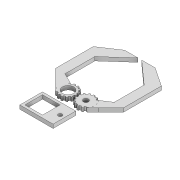
# Autodesk Inventor part: Gripper_dentado
Saved by Autodesk Inventor 2021 (Build 250183000, 183)
## iProperties
Created: 2022-06-07
Part Number: Gripper_dentado
Material: Genérico
Document SubType Name: Modeling
Designer: orgyn
Density: 1 g/cm^3
Appearance: Valor por defecto
Author: orgyn
Autodesk Inventor part; units mm, degrees
ref_plane "YZ Plane" through (0, 0, 0) normal (1, 0, 0) x (0, 1, 0)
ref_plane "XZ Plane" through (0, 0, 0) normal (0, 1, 0) x (-1, 0, 0)
ref_plane "XY Plane" through (0, 0, 0) normal (0, 0, 1) x (1, 0, 0)
sketch "Boceto1" plane through (0, 0, 0) normal (0, 1, 0) x (-1, 0, 0)
  line L0 (6.9821, 0.4997) -> (6.9821, -0.4997)
  line L1 (5.9531, 0.7485) -> (6.9821, 0.4997)
  line L2 (5.9531, -0.7485) -> (6.9821, -0.4997)
  line L3 (5.0388, 3.2574) -> (6.0739, 3.4796)
  line L4 (5.6884, 1.9086) -> (6.5075, 2.5792)
  line L5 (6.0739, 3.4796) -> (6.5075, 2.5792)
  line L6 (3.1265, 5.121) -> (3.9626, 5.7704)
  line L7 (4.2969, 4.1876) -> (4.744, 5.1473)
  line L8 (3.9626, 5.7704) -> (4.744, 5.1473)
  line L9 (0.5949, 5.9704) -> (1.0665, 6.9183)
  line L10 (2.0545, 5.6373) -> (2.0408, 6.6959)
  line L11 (1.0665, 6.9183) -> (2.0408, 6.6959)
  line L12 (-2.0545, 5.6373) -> (-2.0408, 6.6959)
  line L13 (-0.5949, 5.9704) -> (-1.0665, 6.9183)
  line L14 (-2.0408, 6.6959) -> (-1.0665, 6.9183)
  line L15 (-4.2969, 4.1876) -> (-4.744, 5.1473)
  line L16 (-3.1265, 5.121) -> (-3.9626, 5.7704)
  line L17 (-4.744, 5.1473) -> (-3.9626, 5.7704)
  line L18 (-5.6884, 1.9086) -> (-6.5075, 2.5792)
  line L19 (-5.0388, 3.2574) -> (-6.0739, 3.4796)
  line L20 (-6.5075, 2.5792) -> (-6.0739, 3.4796)
  line L21 (-5.9531, -0.7485) -> (-6.9821, -0.4997)
  line L22 (-5.9531, 0.7485) -> (-6.9821, 0.4997)
  line L23 (-6.9821, -0.4997) -> (-6.9821, 0.4997)
  line L24 (-5.0388, -3.2574) -> (-6.0739, -3.4796)
  line L25 (-5.6884, -1.9086) -> (-6.5075, -2.5792)
  line L26 (-6.0739, -3.4796) -> (-6.5075, -2.5792)
  line L27 (-3.1265, -5.121) -> (-3.9626, -5.7704)
  line L28 (-4.2969, -4.1876) -> (-4.744, -5.1473)
  line L29 (-3.9626, -5.7704) -> (-4.744, -5.1473)
  line L30 (-0.5949, -5.9704) -> (-1.0665, -6.9183)
  line L31 (-2.0545, -5.6373) -> (-2.0408, -6.6959)
  line L32 (-1.0665, -6.9183) -> (-2.0408, -6.6959)
  line L33 (2.0545, -5.6373) -> (2.0408, -6.6959)
  line L34 (0.5949, -5.9704) -> (1.0665, -6.9183)
  line L35 (2.0408, -6.6959) -> (1.0665, -6.9183)
  line L36 (4.2969, -4.1876) -> (4.744, -5.1473)
  line L37 (3.1265, -5.121) -> (3.9626, -5.7704)
  line L38 (4.744, -5.1473) -> (3.9626, -5.7704)
  line L39 (5.6884, -1.9086) -> (6.5075, -2.5792)
  line L40 (5.0388, -3.2574) -> (6.0739, -3.4796)
  line L41 (6.5075, -2.5792) -> (6.0739, -3.4796)
  arc A0 (6.5075, 2.5792) -> (6.0739, 3.4796) centre (0, 0) ccw
  arc A1 (4.744, 5.1473) -> (3.9626, 5.7704) centre (0, 0) ccw
  arc A2 (5.9531, 0.7485) -> (5.6884, 1.9086) centre (0, 0) ccw
  arc A3 (5.6884, -1.9086) -> (5.9531, -0.7485) centre (0, 0) ccw
  arc A4 (4.2969, -4.1876) -> (5.0388, -3.2574) centre (0, 0) ccw
  arc A5 (3.9626, -5.7704) -> (4.744, -5.1473) centre (0, 0) ccw
  arc A6 (2.0545, -5.6373) -> (3.1265, -5.121) centre (0, 0) ccw
  arc A7 (1.0665, -6.9183) -> (2.0408, -6.6959) centre (0, 0) ccw
  arc A8 (-0.5949, -5.9704) -> (0.5949, -5.9704) centre (0, 0) ccw
  arc A9 (-2.0408, -6.6959) -> (-1.0665, -6.9183) centre (0, 0) ccw
  arc A10 (-3.1265, -5.121) -> (-2.0545, -5.6373) centre (0, 0) ccw
  arc A11 (-4.744, -5.1473) -> (-3.9626, -5.7704) centre (0, 0) ccw
  arc A12 (-5.0388, -3.2574) -> (-4.2969, -4.1876) centre (0, 0) ccw
  arc A13 (-6.5075, -2.5792) -> (-6.0739, -3.4796) centre (0, 0) ccw
  arc A14 (-5.9531, -0.7485) -> (-5.6884, -1.9086) centre (0, 0) ccw
  arc A15 (-6.9821, 0.4997) -> (-6.9821, -0.4997) centre (0, 0) ccw
  arc A16 (-5.6884, 1.9086) -> (-5.9531, 0.7485) centre (0, 0) ccw
  arc A17 (-6.0739, 3.4796) -> (-6.5075, 2.5792) centre (0, 0) ccw
  arc A18 (-4.2969, 4.1876) -> (-5.0388, 3.2574) centre (0, 0) ccw
  arc A19 (-3.9626, 5.7704) -> (-4.744, 5.1473) centre (0, 0) ccw
  arc A20 (-2.0545, 5.6373) -> (-3.1265, 5.121) centre (0, 0) ccw
  arc A21 (2.0408, 6.6959) -> (1.0665, 6.9183) centre (0, 0) ccw
  arc A22 (-1.0665, 6.9183) -> (-2.0408, 6.6959) centre (0, 0) ccw
  arc A23 (0.5949, 5.9704) -> (-0.5949, 5.9704) centre (0, 0) ccw
  arc A24 (5.0388, 3.2574) -> (4.2969, 4.1876) centre (0, 0) ccw
  arc A25 (3.1265, 5.121) -> (2.0545, 5.6373) centre (0, 0) ccw
  circle A26 centre (0, 0) radius 4.5
  line L42 (-7, 0) -> (-7.2, 0)
  line L43 (-7.2, 0) -> (-21.2, 0)
  line L44 (-7.5804, 2.2898) -> (-7.3217, 1.3245)
  line L45 (-8.6387, 2.2638) -> (-7.5804, 2.2898)
  line L46 (-8.2513, 0.8178) -> (-7.3217, 1.3245)
  line L47 (-10.1712, 4.4505) -> (-9.229, 4.9331)
  line L48 (-9.1947, 3.3158) -> (-8.5771, 4.1756)
  line L49 (-9.229, 4.9331) -> (-8.5771, 4.1756)
  line L50 (-12.5008, 5.7557) -> (-11.8612, 6.5994)
  line L51 (-11.1286, 5.1571) -> (-10.9452, 6.1998)
  line L52 (-11.8612, 6.5994) -> (-10.9452, 6.1998)
  line L53 (-15.1659, 5.921) -> (-14.9557, 6.9586)
  line L54 (-13.6699, 5.977) -> (-13.957, 6.9959)
  line L55 (-17.6388, 4.9135) -> (-17.8996, 5.9395)
  line L56 (-16.3152, 5.613) -> (-17.016, 6.4065)
  line L57 (-19.4297, 2.9328) -> (-20.1098, 3.7441)
  line L58 (-18.5407, 4.1374) -> (-19.5164, 4.5482)
  line L59 (-20.1098, 3.7441) -> (-19.5164, 4.5482)
  line L60 (-20.1838, 0.3713) -> (-21.1486, 0.8071)
  line L61 (-19.9055, 1.8422) -> (-20.9628, 1.789)
  line L62 (-21.1486, 0.8071) -> (-20.9628, 1.789)
  line L63 (-19.7518, -2.2638) -> (-20.8102, -2.2898)
  line L64 (-20.1393, -0.8178) -> (-21.0688, -1.3245)
  line L65 (-20.8102, -2.2898) -> (-21.0688, -1.3245)
  line L66 (-18.2193, -4.4505) -> (-19.1616, -4.9331)
  line L67 (-19.1958, -3.3158) -> (-19.8135, -4.1756)
  line L68 (-19.1616, -4.9331) -> (-19.8135, -4.1756)
  line L69 (-15.8898, -5.7557) -> (-16.5294, -6.5994)
  line L70 (-17.262, -5.1571) -> (-17.4454, -6.1998)
  line L71 (-16.5294, -6.5994) -> (-17.4454, -6.1998)
  line L72 (-13.2247, -5.921) -> (-13.4349, -6.9586)
  line L73 (-14.7207, -5.977) -> (-14.4336, -6.9959)
  line L74 (-13.4349, -6.9586) -> (-14.4336, -6.9959)
  line L75 (-10.7518, -4.9135) -> (-10.491, -5.9395)
  line L76 (-12.0754, -5.613) -> (-11.3745, -6.4065)
  line L77 (-10.491, -5.9395) -> (-11.3745, -6.4065)
  line L78 (-8.9609, -2.9328) -> (-8.2808, -3.7441)
  line L79 (-9.8499, -4.1374) -> (-8.8742, -4.5482)
  line L80 (-8.2808, -3.7441) -> (-8.8742, -4.5482)
  line L81 (-8.2068, -0.3713) -> (-7.242, -0.8071)
  line L82 (-8.4851, -1.8422) -> (-7.4278, -1.789)
  line L83 (-7.242, -0.8071) -> (-7.4278, -1.789)
  arc A27 (-8.5771, 4.1756) -> (-9.229, 4.9331) centre (-14.1953, 0) ccw
  arc A28 (-10.9452, 6.1998) -> (-11.8612, 6.5994) centre (-14.1953, 0) ccw
  arc A29 (-8.6387, 2.2638) -> (-9.1947, 3.3158) centre (-14.1953, 0) ccw
  arc A30 (-8.2068, -0.3713) -> (-8.2513, 0.8178) centre (-14.1953, 0) ccw
  arc A31 (-7.4278, -1.789) -> (-7.242, -0.8071) centre (-14.1953, 0) ccw
  arc A32 (-8.9609, -2.9328) -> (-8.4851, -1.8422) centre (-14.1953, 0) ccw
  arc A33 (-8.8742, -4.5482) -> (-8.2808, -3.7441) centre (-14.1953, 0) ccw
  arc A34 (-10.7518, -4.9135) -> (-9.8499, -4.1374) centre (-14.1953, 0) ccw
  arc A35 (-11.3745, -6.4065) -> (-10.491, -5.9395) centre (-14.1953, 0) ccw
  arc A36 (-13.2247, -5.921) -> (-12.0754, -5.613) centre (-14.1953, 0) ccw
  arc A37 (-14.4336, -6.9959) -> (-13.4349, -6.9586) centre (-14.1953, 0) ccw
  arc A38 (-15.8898, -5.7557) -> (-14.7207, -5.977) centre (-14.1953, 0) ccw
  arc A39 (-17.4454, -6.1998) -> (-16.5294, -6.5994) centre (-14.1953, 0) ccw
  arc A40 (-18.2193, -4.4505) -> (-17.262, -5.1571) centre (-14.1953, 0) ccw
  arc A41 (-19.8135, -4.1756) -> (-19.1616, -4.9331) centre (-14.1953, 0) ccw
  arc A42 (-19.7518, -2.2638) -> (-19.1958, -3.3158) centre (-14.1953, 0) ccw
  arc A43 (-21.0688, -1.3245) -> (-20.8102, -2.2898) centre (-14.1953, 0) ccw
  arc A44 (-20.1838, 0.3713) -> (-20.1393, -0.8178) centre (-14.1953, 0) ccw
  arc A45 (-20.9628, 1.789) -> (-21.1486, 0.8071) centre (-14.1953, 0) ccw
  arc A46 (-19.4297, 2.9328) -> (-19.9055, 1.8422) centre (-14.1953, 0) ccw
  arc A47 (-19.5164, 4.5482) -> (-20.1098, 3.7441) centre (-14.1953, 0) ccw
  arc A48 (-17.6388, 4.9135) -> (-18.5407, 4.1374) centre (-14.1953, 0) ccw
  arc A49 (-13.957, 6.9959) -> (-14.9557, 6.9586) centre (-14.1953, 0) ccw
  arc A50 (-17.016, 6.4065) -> (-17.8996, 5.9395) centre (-14.1953, 0) ccw
  arc A51 (-15.1659, 5.921) -> (-16.3152, 5.613) centre (-14.1953, 0) ccw
  arc A52 (-10.1712, 4.4505) -> (-11.1286, 5.1571) centre (-14.1953, 0) ccw
  arc A53 (-12.5008, 5.7557) -> (-13.6699, 5.977) centre (-14.1953, 0) ccw
  circle A54 centre (-14.1953, 0) radius 2
  line L84 (0, 0) -> (-2, 0)
  line L85 (-2, 0) -> (2, 0)
  line L86 (-14.1953, 0) -> (-16.1953, 0)
  line L87 (0, 0) -> (20, 0)
  line L88 (0, 0) -> (10, 0)
  line L89 (20, -10) -> (10, 0)
  line L90 (20, -40) -> (5, -50)
  line L91 (12.5, -33.8004) -> (12.5, -10)
  line L92 (12.5, -10) -> (4.0311, -2)
  line L93 (10, 0) -> (4.744, 5.1473)
  line L94 (20, -39.7931) -> (20, -10)
  line L95 (12.5, -33.8004) -> (-5.5976, -50)
  line L96 (-34.1953, -10) -> (-24.1953, 0)
  line L97 (-34.1953, -40) -> (-19.1953, -50)
  line L98 (-26.6953, -33.8004) -> (-26.6953, -10)
  line L99 (-24.1953, 0) -> (-19.2423, 4.8505)
  line L100 (-34.1953, -39.7931) -> (-34.1953, -10)
  line L101 (-26.6953, -33.8004) -> (-8.5976, -50)
  line L102 (-26.6953, -10) -> (-18.2193, -4.4505)
  line L103 (-19.3535, -3.0647) -> (-19.0804, -2.8067)
  line L104 (-18.5981, -2.3512) -> (-18.4725, -2.2324)
  line L105 (-18.3019, -2.0713) -> (-18.2264, -2)
  line L106 (5, -50) -> (-5.5976, -50)
  line L107 (-8.5976, -50) -> (-19.1953, -50)
  circle A55 centre (0, 0) radius 4.5
  line L108 (10, 0) -> (4.5, 0)
  line L109 (5.9249, -3.789) -> (8.4708, 1.4976)
  line L110 (5.9249, -3.789) -> (12.5, -10)
  line L111 (12.5, -10) -> (12.5, -33.8004)
  line L112 (12.5, -33.8004) -> (-5.5976, -50)
  line L113 (-5.5976, -50) -> (5, -50)
  line L114 (20, -39.7931) -> (20, -40)
  line L115 (-34.1953, -40) -> (-34.1953, -39.7931)
  line L116 (-19.5164, 4.5482) -> (-19.5334, 4.5655)
  line L117 (12.5, -10) -> (3.9626, -5.7704)
  point P0 (-20.9568, -1.8117)
  point P1 (-18.9393, 5.1473)
  point P2 (5.4573, -3.3472)
  dimension "d14" = 4
  dimension "d6" = 360
  dimension "d9" = 0.2
  dimension "d15" = 2
  dimension "d16" = 4
  constraints: 236 end point, 110 point on circle, 53 centre point, 13 point on line, 5 coincident, 5 horizontal, 3 equal length, 2 horizontal alignment, 2 perpendicular, 2 vertical, 1 midpoint, 106 other
  measures "d9" distance of L42.start L42.end
  measures "d15" distance of L84.start L84.end
  measures "d16" distance of L84.end L85.end
extrude "Extrusión1" add sketch "Boceto1" along normal blind 3 contours L1 A2 L4 A0 L3 A24 L7 L93 L109 L87 L0 | L0 L87 A26 L92 L40 A4 L36 L38 L37 A6 L33 L35 L34 A8 L30 L32 L31 A10 L27 L29 L28 A12 L24 L26 L25 A14 L21 L23 L22 A16 L18 L20 L19 A18 L15 L17 L16 A20 L12 L14 L13 A23 L9 L11 L10 A25 L6 L8 L7 A24 L3 L5 L4 A2 L1 | L87 L109 L39 A3 L2 L0 | L0 L2 A3 L39 L41 L40 L92 A26 L87 | L109 L93 L87 | L87 L89 L94 L114 L90 L106 L95 L91 L92 L109 L41 | A30 L81 L83 L82 A32 L78 L80 L79 A34 L75 L77 L76 A36 L72 L74 L73 A38 L69 L71 L70 A40 L66 L68 L67 A42 L63 L65 L64 A44 L43 A54 | L43 A54 A44 L60 L62 L61 A46 L57 L59 L58 A48 L55 A50 L56 A51 L53 A49 L54 A53 L50 L52 L51 A52 L47 L49 L48 A29 L45 L44 L46 A30 | L92 L117 A5 L36 A4 L40 | L40 L109 L92 | A44 L64 A43 L63 A42 L67 A41 L66 L102 L98 L101 L107 L97 L115 L100 L96 L99 L116 A47 L57 A46 L61 A45 L60
sketch "Boceto2" plane through (0, 0, 0) normal (0, -1, 0) x (1, 0, 0)
  line L0 (0, 0) -> (0, 20.3173)
  line L1 (0, 20.3173) -> (14, 20.3173)
  line L2 (0, 20.3173) -> (0, 13.3173)
  line L3 (0, 13.3173) -> (-7, 13.3173)
  line L4 (-7, 13.3173) -> (-7, 27.3173)
  line L5 (-7, 27.3173) -> (7, 27.3173)
  line L6 (7, 27.3173) -> (7, 13.3173)
  line L7 (7, 13.3173) -> (0, 13.3173)
  circle A0 centre (14, 20.3173) radius 1.5
  line L8 (-7, 20.3173) -> (-9, 20.3173)
  line L9 (-9, 20.3173) -> (-9, 11.3173)
  line L10 (-9, 11.3173) -> (19.3488, 11.3173)
  line L11 (-9, 20.3173) -> (-9, 29.3173)
  line L12 (-9, 29.3173) -> (21.7108, 29.3173)
  line L13 (17.4066, 11.3173) -> (17.4066, 29.3173)
  dimension "d26" = 14
  dimension "d27" = 7
  dimension "d28" = 7
  dimension "d29" = 14
  dimension "d30" = 14
  dimension "d31" = 14
  dimension "d32" = 3
  dimension "d33" = 2
  dimension "d34" = 9
  dimension "d35" = 9
  constraints: 28 end point, 8 perpendicular, 4 point on line, 2 horizontal, 2 vertical, 1 centre point, 1 coincident, 1 midpoint
  measures "d26" distance of L0.end L1.end
  measures "d27" distance of L0.end L2.end
  measures "d28" distance of L2.end L3.end
  measures "d29" distance of L3.end L4.end
  measures "d30" distance of L4.end L5.end
  measures "d31" distance of L5.end L6.end
  measures "d32" diameter of A0
  measures "d33" distance of L8.start L8.end
  measures "d34" distance of L8.end L9.end
  measures "d35" distance of L8.end L11.end
extrude "Extrusión2" add sketch "Boceto2" against normal blind 3 contours L7 L6 L5 L4 L8 L11 L12 L13 L10 L0 | L0 L10 L9 L8 L4 L3
